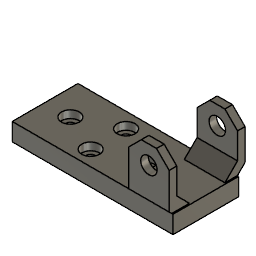
cnc head cable chain (Autodesk Fusion 360 design; units mm, degrees)
Autodesk Fusion 360 part; units mm, degrees
sketch "Szkic1" plane through (0, 0, 0) normal (0, 0, 1) x (1, 0, 0)
  line L0 (-38.5, -13) -> (38.5, -13)
  line L1 (38.5, -13) -> (38.5, 13)
  line L2 (38.5, 13) -> (-38.5, 13)
  line L3 (-38.5, 13) -> (-38.5, -13)
  circle A0 centre (-15, 0) radius 1.75
  circle A1 centre (0, 7) radius 1.75
  circle A2 centre (15, 0) radius 1.75
  circle A3 centre (0, -7) radius 1.75
  circle A4 centre (0, 7) radius 3.5
  circle A5 centre (0, -7) radius 3.5
  circle A6 centre (15, 0) radius 3.5
  circle A7 centre (-15, 0) radius 3.5
  line L4 (-25, 13) -> (25, 13)
  line L5 (25, -13) -> (-25, -13)
  line L6 (-25, -13) -> (-25, 13)
  line L7 (22, 13) -> (38, 13)
  line L8 (38, 13) -> (38, -11)
  line L9 (38, -11) -> (22, -11)
  line L10 (22, -11) -> (22, 13)
  dimension "d1" = 3.5
  dimension "d3" = 3.5
  dimension "d4" = 3.5
  dimension "d5" = 3.5
  dimension "d6" = 7
  dimension "d7" = 7
  dimension "d8" = 7
  dimension "d9" = 7
  constraint concentric A1 A4
  constraint concentric A3 A5
  constraint concentric A2 A6
  constraint concentric A0 A7
  constraint parallel L4 L5
  constraint coincident L2 L4.end
  constraint coincident L2 L4.start
  constraint perpendicular L7 L8
  constraint parallel L7 L9
  constraint parallel L8 L10
  constraint coincident L2 L7.end
  constraint coincident L2 L7.start
  measures "d1" diameter of A0
  measures "d3" diameter of A1
  measures "d4" diameter of A2
  measures "d5" diameter of A3
  measures "d6" diameter of A4
  measures "d7" diameter of A5
  measures "d8" diameter of A6
  measures "d9" diameter of A7
extrude "Wyciągnięcie proste1" add sketch "Szkic1" along normal blind 7 contours L0 L1 L2 L4 L5 L6 L8 L9 L10
extrude "Wyciągnięcie proste2" add sketch "Szkic1" along normal blind 4 contours A4 | A5 | A6 | A7
extrude "Wyciągnięcie proste3" add sketch "Szkic1" along normal blind 28 contours L2 L4 L7 L8 L9 L10
sketch "Szkic2" plane through (0, -11, 0) normal (0, -1, 0) x (1, 0, 0)
  line L0 (22, 7) -> (38, 7)
  line L1 (38, 7) -> (38, 28)
  line L2 (38, 28) -> (22, 28)
  line L3 (22, 28) -> (22, 7)
  circle A0 centre (30, 20) radius 3.25
  dimension "d16" = 6.5
  measures "d16" diameter of A0
extrude "Wyciągnięcie proste4" add sketch "Szkic2" along normal blind 3
extrude "Wyciągnięcie proste5" cut 1 faces at (29.218, -11, 19.4246) along direction (0, 1, 0) blind 91
sketch "Szkic3" plane through (0, 13, 0) normal (0, 1, 0) x (-1, 0, 0)
  circle A0 centre (-30, 20) radius 3.25
  line L0 (-38.5, 0) -> (25, 0)
  line L1 (25, 0) -> (25, 7)
  line L2 (25, 7) -> (-22, 7)
  line L3 (-22, 7) -> (-22, 28)
  line L4 (-22, 28) -> (-38, 28)
  line L5 (-38, 28) -> (-38, 7)
  line L6 (-38, 7) -> (-38.5, 7)
  line L7 (-38.5, 7) -> (-38.5, 0)
  line L8 (-38, 28) -> (-22, 28)
  line L9 (-22, 28) -> (-22, 7)
  line L10 (-22, 7) -> (-38, 7)
  line L11 (-38, 7) -> (-38, 28)
  constraint perpendicular L8 L9
  constraint parallel L8 L10
  constraint parallel L9 L11
  constraint coincident L3.end L4.start
  constraint perpendicular L3 L8
  constraint coincident L4.end L5.start
extrude "Wyciągnięcie proste6" add sketch "Szkic3" along normal blind 3 contours L3 L4 L5 L8 L9 L10 L11
extrude "Wyciągnięcie proste7" cut sketch "Szkic3" against normal blind 24 contours L3 L4 L5 L8 L9 L10 L11
chamfer "Fazowanie1" distance 6 angle 45 1 edges at (30, -11, 7)
chamfer "Fazowanie2" distance 2.99 angle 45 1 edges at (30, 16, 7)
delete_face "Usuń powierzchnię1" 1 faces at (27.3333, -9, 11)
chamfer "Fazowanie3" distance 1 angle 45 1 edges at (30, -14, 7)
chamfer "Fazowanie4" distance 5 angle 45 1 edges at (30, -11, 7)
extrude "Wyciągnięcie proste8" add 1 faces at (11.8333, 13, 2.3333) along direction (0, 1, 0) blind 1
chamfer "Fazowanie5" distance 5 angle 45 1 edges at (30, 13, 7)
extrude "Wyciągnięcie proste9" cut 1 faces at (17.1667, 14, 2.3333) along direction (0, -1, 0) blind 1
extrude "Wyciągnięcie proste10" cut 2 faces at (27.3333, -13, 28) (27.3333, 14, 28) along direction (0, 0, -1) blind 0.75
chamfer "Fazowanie6" distance 5 angle 45 2 edges at (38, -12.5, 27.25) (38, 14.5, 27.25)
chamfer "Fazowanie7" distance 5 angle 45 2 edges at (22, 14.5, 27.25) (22, -12.5, 27.25)
